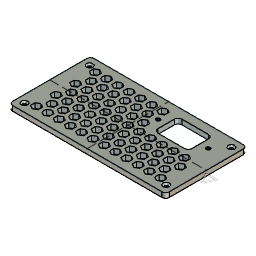
SFX+HDPLEX+Plate (Autodesk Fusion 360 design; units mm, degrees)
part number: 2025-09-21-12-47-08-713
Autodesk Fusion 360 part; units mm, degrees
sketch "Sketch1" plane through (0, 0, 0) normal (0, 0, 1) x (1, 0, 0)
  line L0 (59.5, 32.5) -> (-59.5, 32.5)
  line L1 (-62.5, 29.5) -> (-62.5, -29.5)
  line L2 (-59.5, -32.5) -> (59.5, -32.5)
  line L3 (62.5, -29.5) -> (62.5, 29.5)
  line L4 (62.5, 32.5) -> (-62.5, -32.5) construction
  line L5 (-62.5, 32.5) -> (62.5, -32.5) construction
  arc A0 (-59.5, 32.5) -> (-62.5, 29.5) centre (-59.5, 29.5) ccw
  arc A1 (62.5, 29.5) -> (59.5, 32.5) centre (59.5, 29.5) ccw
  arc A2 (-62.5, -29.5) -> (-59.5, -32.5) centre (-59.5, -29.5) ccw
  arc A3 (59.5, -32.5) -> (62.5, -29.5) centre (59.5, -29.5) ccw
  dimension "d1" = 125
  dimension "d2" = 65
  dimension "d3" = 3
  dimension "d4" = 3
  dimension "d5" = 3
  dimension "d6" = 3
  constraint horizontal L0
  constraint perpendicular L0 L1
  constraint parallel L0 L2
  constraint parallel L1 L3
  constraint coincident L4 origin
  constraint coincident L5 origin
  constraint coincident L5.start L1
  constraint coincident L5.start L0
  constraint tangent L1 A0
  constraint tangent L0 A0
  constraint coincident L4.start L0
  constraint coincident L4.start L3
  constraint tangent L0 A1
  constraint tangent L3 A1
  constraint coincident L4.end L1
  constraint coincident L4.end L2
  constraint tangent L1 A2
  constraint tangent L2 A2
  constraint coincident L5.end L2
  constraint coincident L5.end L3
  constraint tangent L2 A3
  constraint tangent L3 A3
  measures "d1" distance of L4.end L5.end
  measures "d2" distance of L5.start L4.end
  measures "d3" radius of A0
  measures "d4" radius of A1
  measures "d5" radius of A2
  measures "d6" radius of A3
extrude "Extrude1" add sketch "Sketch1" along normal blind 4
sketch "Sketch2" plane through (0, 0, 4) normal (0, 0, 1) x (-1, 0, 0)
  arc A0 (-59.5, 32.5) -> (-62.5, 29.5) centre (-59.5, 29.5) ccw
  line L0 (-62.5, 29.5) -> (-62.5, -29.5)
  arc A1 (-62.5, -29.5) -> (-59.5, -32.5) centre (-59.5, -29.5) ccw
  line L1 (-59.5, -32.5) -> (59.5, -32.5)
  arc A2 (59.5, -32.5) -> (62.5, -29.5) centre (59.5, -29.5) ccw
  line L2 (62.5, -29.5) -> (62.5, 29.5)
  arc A3 (62.5, 29.5) -> (59.5, 32.5) centre (59.5, 29.5) ccw
  line L3 (59.5, 32.5) -> (-59.5, 32.5)
  line L4 (0, 32.5) -> (0, -32.5) construction
  line L5 (62.5, 0) -> (-62.5, 0) construction
  constraint midpoint L3 L4.start
  constraint midpoint L1 L4.end
  constraint midpoint L2 L5.start
  constraint midpoint L0 L5.end
sketch "Sketch3" plane through (0, 0, 4) normal (0, 0, 1) x (1, 0, 0)
  line L0 (-62.5, 0) -> (62.5, 0)
  line L1 (0, -32.5) -> (0, 32.5)
  circle A0 centre (-56.5, -26) radius 1.75
  circle A1 centre (-56.5, 26) radius 1.75
  circle A2 centre (56.5, 26) radius 1.75
  circle A3 centre (56.5, -26) radius 1.75
  point P0 (-56.5, 26)
  point P1 (56.5, 26)
  point P2 (56.5, -26)
  point P3 (-56.5, -26)
  dimension "d10" = 56.5
  dimension "d11" = 26
  dimension "d12" = 56.5
  dimension "d13" = 26
  dimension "d14" = 56.5
  dimension "d15" = 26
  dimension "d17" = 26
  dimension "d18" = 56.5
  dimension "d19" = 3.5
  dimension "d20" = 3.5
  dimension "d21" = 3.5
  dimension "d22" = 3.5
  constraint coincident P3 A0.centre
  constraint coincident P0 A1.centre
  constraint coincident P1 A2.centre
  constraint coincident P2 A3.centre
  measures "d10" distance of P0 L1
  measures "d11" distance of P0 L0
  measures "d12" distance of L1 P1
  measures "d13" distance of L0 P1
  measures "d14" distance of L1 P2
  measures "d15" distance of L0 P2
  measures "d17" distance of L0 P3
  measures "d18" distance of L1 P3
  measures "d19" diameter of A0
  measures "d20" diameter of A1
  measures "d21" diameter of A2
  measures "d22" diameter of A3
hole "Hole1" at (-56.5, 26, 4) at (-56.5, -26, 4) at (56.5, 26, 4) at (56.5, -26, 4) direction (0, 0, -1) diameter 2.529 depth 4 tip angle 118 countersink diameter 5 countersink angle 90
thread "Thread1" "ISO Metric profile 3.0 M3x0.5 M3x0.5 6H" thread offset 0 thread depth 7.4
sketch "Sketch4" plane through (0, 0, 4) normal (0, 0, 1) x (-1, 0, 0)
  line L0 (-17.4, -25.6) -> (-38.6, -25.6)
  line L1 (-41.6, -22.6) -> (-41.6, -9.4)
  line L2 (-38.6, -6.4) -> (-17.4, -6.4)
  line L3 (-14.4, -9.4) -> (-14.4, -22.6)
  arc A0 (-17.4, -25.6) -> (-14.4, -22.6) centre (-17.4, -22.6) ccw
  arc A1 (-41.6, -22.6) -> (-38.6, -25.6) centre (-38.6, -22.6) ccw
  arc A2 (-14.4, -9.4) -> (-17.4, -6.4) centre (-17.4, -9.4) ccw
  arc A3 (-38.6, -6.4) -> (-41.6, -9.4) centre (-38.6, -9.4) ccw
  line L4 (0, 32.5) -> (0, -32.5)
  line L5 (62.5, 0) -> (-62.5, 0)
  circle A4 centre (-48, -16) radius 1
  circle A5 centre (-8, -16) radius 1
  point P0 (-14.4, -25.6)
  point P1 (-41.6, -25.6)
  point P2 (-14.4, -6.4)
  point P3 (-48, -16)
  point P4 (-8, -16)
  point P5 (-48, -16)
  dimension "d32" = 3
  dimension "d33" = 3
  dimension "d34" = 3
  dimension "d35" = 3
  dimension "d40" = 2
  dimension "d41" = 2
  constraint coincident P0 L3
  constraint coincident P0 L0
  constraint tangent L3 A0
  constraint tangent L0 A0
  constraint coincident P1 L0
  constraint coincident P1 L1
  constraint tangent L0 A1
  constraint tangent L1 A1
  constraint coincident P2 L2
  constraint coincident P2 L3
  constraint tangent L2 A2
  constraint tangent L3 A2
  constraint tangent L2 A3
  constraint tangent L1 A3
  constraint coincident P5 P3
  constraint coincident P4 A5.centre
  measures "d32" radius of A0
  measures "d33" radius of A1
  measures "d34" radius of A2
  measures "d35" radius of A3
  measures "d40" diameter of A4
  measures "d41" diameter of A5
extrude "Extrude2" cut sketch "Sketch4" against normal blind 4
sketch "Sketch5" plane through (0, 0, 4) normal (0, 0, 1) x (-1, 0, 0)
  point P0 (-48, -16)
  point P1 (-8, -16)
hole "Hole2" at (48, 16, 4) at (8, 16, 4) direction (0, 0, -1) diameter 2.529 depth 4 tip angle 118
thread "Thread2" "ISO Metric profile 3.0 M3x0.5 M3x0.5 6H" thread offset 0 thread depth 7.4
sketch "Sketch6" plane through (0, 0, 4) normal (0, 0, 1) x (-1, 0, 0)
  line L0 (-3, -1.7321) -> (0, -3.4641)
  line L1 (0, -3.4641) -> (3, -1.7321)
  line L2 (3, -1.7321) -> (3, 1.7321)
  line L3 (3, 1.7321) -> (0, 3.4641)
  line L4 (0, 3.4641) -> (-3, 1.7321)
  line L5 (-3, 1.7321) -> (-3, -1.7321)
  line L6 (-48, -1.7321) -> (-45, -3.4641)
  line L7 (-45, -3.4641) -> (-42, -1.7321)
  line L8 (-42, -1.7321) -> (-42, 1.7321)
  line L9 (-42, 1.7321) -> (-45, 3.4641)
  line L10 (-48, 1.7321) -> (-48, -1.7321)
  line L11 (-45, 3.4641) -> (-48, 1.7321)
  line L12 (-39, -1.7321) -> (-36, -3.4641)
  line L13 (-36, -3.4641) -> (-33, -1.7321)
  line L14 (-33, -1.7321) -> (-33, 1.7321)
  line L15 (-33, 1.7321) -> (-36, 3.4641)
  line L16 (-39, 1.7321) -> (-39, -1.7321)
  line L17 (-36, 3.4641) -> (-39, 1.7321)
  line L18 (-30, -1.7321) -> (-27, -3.4641)
  line L19 (-27, -3.4641) -> (-24, -1.7321)
  line L20 (-24, -1.7321) -> (-24, 1.7321)
  line L21 (-24, 1.7321) -> (-27, 3.4641)
  line L22 (-30, 1.7321) -> (-30, -1.7321)
  line L23 (-27, 3.4641) -> (-30, 1.7321)
  line L24 (-21, -1.7321) -> (-18, -3.4641)
  line L25 (-18, -3.4641) -> (-15, -1.7321)
  line L26 (-15, -1.7321) -> (-15, 1.7321)
  line L27 (-15, 1.7321) -> (-18, 3.4641)
  line L28 (-21, 1.7321) -> (-21, -1.7321)
  line L29 (-18, 3.4641) -> (-21, 1.7321)
  line L30 (-12, -1.7321) -> (-9, -3.4641)
  line L31 (-9, -3.4641) -> (-6, -1.7321)
  line L32 (-6, -1.7321) -> (-6, 1.7321)
  line L33 (-6, 1.7321) -> (-9, 3.4641)
  line L34 (-12, 1.7321) -> (-12, -1.7321)
  line L35 (-9, 3.4641) -> (-12, 1.7321)
  line L36 (6, -1.7321) -> (9, -3.4641)
  line L37 (9, -3.4641) -> (12, -1.7321)
  line L38 (12, -1.7321) -> (12, 1.7321)
  line L39 (12, 1.7321) -> (9, 3.4641)
  line L40 (6, 1.7321) -> (6, -1.7321)
  line L41 (9, 3.4641) -> (6, 1.7321)
  line L42 (15, -1.7321) -> (18, -3.4641)
  line L43 (18, -3.4641) -> (21, -1.7321)
  line L44 (21, -1.7321) -> (21, 1.7321)
  line L45 (21, 1.7321) -> (18, 3.4641)
  line L46 (15, 1.7321) -> (15, -1.7321)
  line L47 (18, 3.4641) -> (15, 1.7321)
  line L48 (24, -1.7321) -> (27, -3.4641)
  line L49 (27, -3.4641) -> (30, -1.7321)
  line L50 (30, -1.7321) -> (30, 1.7321)
  line L51 (30, 1.7321) -> (27, 3.4641)
  line L52 (24, 1.7321) -> (24, -1.7321)
  line L53 (27, 3.4641) -> (24, 1.7321)
  line L54 (33, -1.7321) -> (36, -3.4641)
  line L55 (36, -3.4641) -> (39, -1.7321)
  line L56 (39, -1.7321) -> (39, 1.7321)
  line L57 (39, 1.7321) -> (36, 3.4641)
  line L58 (33, 1.7321) -> (33, -1.7321)
  line L59 (36, 3.4641) -> (33, 1.7321)
  line L60 (42, -1.7321) -> (45, -3.4641)
  line L61 (45, -3.4641) -> (48, -1.7321)
  line L62 (48, -1.7321) -> (48, 1.7321)
  line L63 (48, 1.7321) -> (45, 3.4641)
  line L64 (42, 1.7321) -> (42, -1.7321)
  line L65 (45, 3.4641) -> (42, 1.7321)
  line L66 (48, -1.7321) -> (48, 1.7321)
  line L67 (48, 1.7321) -> (45, 3.4641)
  line L68 (45, 3.4641) -> (42, 1.7321)
  line L69 (42, 1.7321) -> (42, -1.7321)
  line L70 (42, -1.7321) -> (45, -3.4641)
  line L71 (45, -3.4641) -> (48, -1.7321)
  line L72 (39, -1.7321) -> (39, 1.7321)
  line L73 (39, 1.7321) -> (36, 3.4641)
  line L74 (36, 3.4641) -> (33, 1.7321)
  line L75 (33, 1.7321) -> (33, -1.7321)
  line L76 (36, -3.4641) -> (39, -1.7321)
  line L77 (33, -1.7321) -> (36, -3.4641)
  line L78 (30, -1.7321) -> (30, 1.7321)
  line L79 (30, 1.7321) -> (27, 3.4641)
  line L80 (27, 3.4641) -> (24, 1.7321)
  line L81 (24, 1.7321) -> (24, -1.7321)
  line L82 (27, -3.4641) -> (30, -1.7321)
  line L83 (24, -1.7321) -> (27, -3.4641)
  line L84 (21, -1.7321) -> (21, 1.7321)
  line L85 (21, 1.7321) -> (18, 3.4641)
  line L86 (18, 3.4641) -> (15, 1.7321)
  line L87 (15, 1.7321) -> (15, -1.7321)
  line L88 (18, -3.4641) -> (21, -1.7321)
  line L89 (15, -1.7321) -> (18, -3.4641)
  line L90 (12, -1.7321) -> (12, 1.7321)
  line L91 (12, 1.7321) -> (9, 3.4641)
  line L92 (9, 3.4641) -> (6, 1.7321)
  line L93 (6, 1.7321) -> (6, -1.7321)
  line L94 (9, -3.4641) -> (12, -1.7321)
  line L95 (6, -1.7321) -> (9, -3.4641)
  line L96 (3, -1.7321) -> (3, 1.7321)
  line L97 (3, 1.7321) -> (0, 3.4641)
  line L98 (0, 3.4641) -> (-3, 1.7321)
  line L99 (-3, 1.7321) -> (-3, -1.7321)
  line L100 (0, -3.4641) -> (3, -1.7321)
  line L101 (-3, -1.7321) -> (0, -3.4641)
  line L102 (-6, -1.7321) -> (-6, 1.7321)
  line L103 (-6, 1.7321) -> (-9, 3.4641)
  line L104 (-9, 3.4641) -> (-12, 1.7321)
  line L105 (-12, 1.7321) -> (-12, -1.7321)
  line L106 (-9, -3.4641) -> (-6, -1.7321)
  line L107 (-12, -1.7321) -> (-9, -3.4641)
  line L108 (-15, -1.7321) -> (-15, 1.7321)
  line L109 (-15, 1.7321) -> (-18, 3.4641)
  line L110 (-18, 3.4641) -> (-21, 1.7321)
  line L111 (-21, 1.7321) -> (-21, -1.7321)
  line L112 (-18, -3.4641) -> (-15, -1.7321)
  line L113 (-21, -1.7321) -> (-18, -3.4641)
  line L114 (-24, -1.7321) -> (-24, 1.7321)
  line L115 (-24, 1.7321) -> (-27, 3.4641)
  line L116 (-27, 3.4641) -> (-30, 1.7321)
  line L117 (-30, 1.7321) -> (-30, -1.7321)
  line L118 (-27, -3.4641) -> (-24, -1.7321)
  line L119 (-30, -1.7321) -> (-27, -3.4641)
  line L120 (-33, -1.7321) -> (-33, 1.7321)
  line L121 (-33, 1.7321) -> (-36, 3.4641)
  line L122 (-36, 3.4641) -> (-39, 1.7321)
  line L123 (-39, 1.7321) -> (-39, -1.7321)
  line L124 (-36, -3.4641) -> (-33, -1.7321)
  line L125 (-39, -1.7321) -> (-36, -3.4641)
  line L126 (-42, -1.7321) -> (-42, 1.7321)
  line L127 (-42, 1.7321) -> (-45, 3.4641)
  line L128 (-45, 3.4641) -> (-48, 1.7321)
  line L129 (-48, 1.7321) -> (-48, -1.7321)
  line L130 (-45, -3.4641) -> (-42, -1.7321)
  line L131 (-48, -1.7321) -> (-45, -3.4641)
  line L132 (48, -1.7321) -> (48, 1.7321)
  line L133 (48, 1.7321) -> (45, 3.4641)
  line L134 (45, 3.4641) -> (42, 1.7321)
  line L135 (42, 1.7321) -> (42, -1.7321)
  line L136 (42, -1.7321) -> (45, -3.4641)
  line L137 (45, -3.4641) -> (48, -1.7321)
  line L138 (39, -1.7321) -> (39, 1.7321)
  line L139 (39, 1.7321) -> (36, 3.4641)
  line L140 (36, 3.4641) -> (33, 1.7321)
  line L141 (33, 1.7321) -> (33, -1.7321)
  line L142 (36, -3.4641) -> (39, -1.7321)
  line L143 (33, -1.7321) -> (36, -3.4641)
  line L144 (30, -1.7321) -> (30, 1.7321)
  line L145 (30, 1.7321) -> (27, 3.4641)
  line L146 (27, 3.4641) -> (24, 1.7321)
  line L147 (24, 1.7321) -> (24, -1.7321)
  line L148 (27, -3.4641) -> (30, -1.7321)
  line L149 (24, -1.7321) -> (27, -3.4641)
  line L150 (21, -1.7321) -> (21, 1.7321)
  line L151 (21, 1.7321) -> (18, 3.4641)
  line L152 (18, 3.4641) -> (15, 1.7321)
  line L153 (15, 1.7321) -> (15, -1.7321)
  line L154 (18, -3.4641) -> (21, -1.7321)
  line L155 (15, -1.7321) -> (18, -3.4641)
  line L156 (12, -1.7321) -> (12, 1.7321)
  line L157 (12, 1.7321) -> (9, 3.4641)
  line L158 (9, 3.4641) -> (6, 1.7321)
  line L159 (6, 1.7321) -> (6, -1.7321)
  line L160 (9, -3.4641) -> (12, -1.7321)
  line L161 (6, -1.7321) -> (9, -3.4641)
  line L162 (3, -1.7321) -> (3, 1.7321)
  line L163 (3, 1.7321) -> (0, 3.4641)
  line L164 (0, 3.4641) -> (-3, 1.7321)
  line L165 (-3, 1.7321) -> (-3, -1.7321)
  line L166 (0, -3.4641) -> (3, -1.7321)
  line L167 (-3, -1.7321) -> (0, -3.4641)
  line L168 (-6, -1.7321) -> (-6, 1.7321)
  line L169 (-6, 1.7321) -> (-9, 3.4641)
  line L170 (-9, 3.4641) -> (-12, 1.7321)
  line L171 (-12, 1.7321) -> (-12, -1.7321)
  line L172 (-9, -3.4641) -> (-6, -1.7321)
  line L173 (-12, -1.7321) -> (-9, -3.4641)
  line L174 (-15, -1.7321) -> (-15, 1.7321)
  line L175 (-15, 1.7321) -> (-18, 3.4641)
  line L176 (-18, 3.4641) -> (-21, 1.7321)
  line L177 (-21, 1.7321) -> (-21, -1.7321)
  line L178 (-18, -3.4641) -> (-15, -1.7321)
  line L179 (-21, -1.7321) -> (-18, -3.4641)
  line L180 (-24, -1.7321) -> (-24, 1.7321)
  line L181 (-24, 1.7321) -> (-27, 3.4641)
  line L182 (-27, 3.4641) -> (-30, 1.7321)
  line L183 (-30, 1.7321) -> (-30, -1.7321)
  line L184 (-27, -3.4641) -> (-24, -1.7321)
  line L185 (-30, -1.7321) -> (-27, -3.4641)
  line L186 (-33, -1.7321) -> (-33, 1.7321)
  line L187 (-33, 1.7321) -> (-36, 3.4641)
  line L188 (-36, 3.4641) -> (-39, 1.7321)
  line L189 (-39, 1.7321) -> (-39, -1.7321)
  line L190 (-36, -3.4641) -> (-33, -1.7321)
  line L191 (-39, -1.7321) -> (-36, -3.4641)
  line L192 (-42, -1.7321) -> (-42, 1.7321)
  line L193 (-42, 1.7321) -> (-45, 3.4641)
  line L194 (-45, 3.4641) -> (-48, 1.7321)
  line L195 (-48, 1.7321) -> (-48, -1.7321)
  line L196 (-45, -3.4641) -> (-42, -1.7321)
  line L197 (-48, -1.7321) -> (-45, -3.4641)
  line L198 (48, -1.7321) -> (48, 1.7321)
  line L199 (48, 1.7321) -> (45, 3.4641)
  line L200 (45, 3.4641) -> (42, 1.7321)
  line L201 (42, 1.7321) -> (42, -1.7321)
  line L202 (42, -1.7321) -> (45, -3.4641)
  line L203 (45, -3.4641) -> (48, -1.7321)
  line L204 (39, -1.7321) -> (39, 1.7321)
  line L205 (39, 1.7321) -> (36, 3.4641)
  line L206 (36, 3.4641) -> (33, 1.7321)
  line L207 (33, 1.7321) -> (33, -1.7321)
  line L208 (36, -3.4641) -> (39, -1.7321)
  line L209 (33, -1.7321) -> (36, -3.4641)
  line L210 (30, -1.7321) -> (30, 1.7321)
  line L211 (30, 1.7321) -> (27, 3.4641)
  line L212 (27, 3.4641) -> (24, 1.7321)
  line L213 (24, 1.7321) -> (24, -1.7321)
  line L214 (27, -3.4641) -> (30, -1.7321)
  line L215 (24, -1.7321) -> (27, -3.4641)
  line L216 (21, -1.7321) -> (21, 1.7321)
  line L217 (21, 1.7321) -> (18, 3.4641)
  line L218 (18, 3.4641) -> (15, 1.7321)
  line L219 (15, 1.7321) -> (15, -1.7321)
  line L220 (18, -3.4641) -> (21, -1.7321)
  line L221 (15, -1.7321) -> (18, -3.4641)
  line L222 (12, -1.7321) -> (12, 1.7321)
  line L223 (12, 1.7321) -> (9, 3.4641)
  line L224 (9, 3.4641) -> (6, 1.7321)
  line L225 (6, 1.7321) -> (6, -1.7321)
  line L226 (9, -3.4641) -> (12, -1.7321)
  line L227 (6, -1.7321) -> (9, -3.4641)
  line L228 (3, -1.7321) -> (3, 1.7321)
  line L229 (3, 1.7321) -> (0, 3.4641)
  line L230 (0, 3.4641) -> (-3, 1.7321)
  line L231 (-3, 1.7321) -> (-3, -1.7321)
  line L232 (0, -3.4641) -> (3, -1.7321)
  line L233 (-3, -1.7321) -> (0, -3.4641)
  line L234 (-6, -1.7321) -> (-6, 1.7321)
  line L235 (-6, 1.7321) -> (-9, 3.4641)
  line L236 (-9, 3.4641) -> (-12, 1.7321)
  line L237 (-12, 1.7321) -> (-12, -1.7321)
  line L238 (-9, -3.4641) -> (-6, -1.7321)
  line L239 (-12, -1.7321) -> (-9, -3.4641)
  line L240 (-15, -1.7321) -> (-15, 1.7321)
  line L241 (-15, 1.7321) -> (-18, 3.4641)
  line L242 (-18, 3.4641) -> (-21, 1.7321)
  line L243 (-21, 1.7321) -> (-21, -1.7321)
  line L244 (-18, -3.4641) -> (-15, -1.7321)
  line L245 (-21, -1.7321) -> (-18, -3.4641)
  line L246 (-24, -1.7321) -> (-24, 1.7321)
  line L247 (-24, 1.7321) -> (-27, 3.4641)
  line L248 (-27, 3.4641) -> (-30, 1.7321)
  line L249 (-30, 1.7321) -> (-30, -1.7321)
  line L250 (-27, -3.4641) -> (-24, -1.7321)
  line L251 (-30, -1.7321) -> (-27, -3.4641)
  line L252 (-33, -1.7321) -> (-33, 1.7321)
  line L253 (-33, 1.7321) -> (-36, 3.4641)
  line L254 (-36, 3.4641) -> (-39, 1.7321)
  line L255 (-39, 1.7321) -> (-39, -1.7321)
  line L256 (-36, -3.4641) -> (-33, -1.7321)
  line L257 (-39, -1.7321) -> (-36, -3.4641)
  line L258 (-42, -1.7321) -> (-42, 1.7321)
  line L259 (-42, 1.7321) -> (-45, 3.4641)
  line L260 (-45, 3.4641) -> (-48, 1.7321)
  line L261 (-48, 1.7321) -> (-48, -1.7321)
  line L262 (-45, -3.4641) -> (-42, -1.7321)
  line L263 (-48, -1.7321) -> (-45, -3.4641)
  line L264 (-30, 1.7321) -> (-30, -1.7321)
  line L265 (-30, -1.7321) -> (-27, -3.4641)
  line L266 (-27, -3.4641) -> (-24, -1.7321)
  line L267 (-24, -1.7321) -> (-24, 1.7321)
  line L268 (-27, 3.4641) -> (-30, 1.7321)
  line L269 (-24, 1.7321) -> (-27, 3.4641)
  line L270 (-39, 1.7321) -> (-39, -1.7321)
  line L271 (-39, -1.7321) -> (-36, -3.4641)
  line L272 (-36, -3.4641) -> (-33, -1.7321)
  line L273 (-33, -1.7321) -> (-33, 1.7321)
  line L274 (-36, 3.4641) -> (-39, 1.7321)
  line L275 (-33, 1.7321) -> (-36, 3.4641)
  line L276 (-48, 1.7321) -> (-48, -1.7321)
  line L277 (-48, -1.7321) -> (-45, -3.4641)
  line L278 (-45, -3.4641) -> (-42, -1.7321)
  line L279 (-42, -1.7321) -> (-42, 1.7321)
  line L280 (-45, 3.4641) -> (-48, 1.7321)
  line L281 (-42, 1.7321) -> (-45, 3.4641)
  line L282 (-21, 1.7321) -> (-21, -1.7321)
  line L283 (-21, -1.7321) -> (-18, -3.4641)
  line L284 (-18, -3.4641) -> (-15, -1.7321)
  line L285 (-15, -1.7321) -> (-15, 1.7321)
  line L286 (-18, 3.4641) -> (-21, 1.7321)
  line L287 (-15, 1.7321) -> (-18, 3.4641)
  line L288 (-12, 1.7321) -> (-12, -1.7321)
  line L289 (-12, -1.7321) -> (-9, -3.4641)
  line L290 (-9, -3.4641) -> (-6, -1.7321)
  line L291 (-6, -1.7321) -> (-6, 1.7321)
  line L292 (-9, 3.4641) -> (-12, 1.7321)
  line L293 (-6, 1.7321) -> (-9, 3.4641)
  line L294 (-3, 1.7321) -> (-3, -1.7321)
  line L295 (-3, -1.7321) -> (0, -3.4641)
  line L296 (0, -3.4641) -> (3, -1.7321)
  line L297 (3, -1.7321) -> (3, 1.7321)
  line L298 (0, 3.4641) -> (-3, 1.7321)
  line L299 (3, 1.7321) -> (0, 3.4641)
  line L300 (6, 1.7321) -> (6, -1.7321)
  line L301 (6, -1.7321) -> (9, -3.4641)
  line L302 (9, -3.4641) -> (12, -1.7321)
  line L303 (12, -1.7321) -> (12, 1.7321)
  line L304 (9, 3.4641) -> (6, 1.7321)
  line L305 (12, 1.7321) -> (9, 3.4641)
  line L306 (15, 1.7321) -> (15, -1.7321)
  line L307 (15, -1.7321) -> (18, -3.4641)
  line L308 (18, -3.4641) -> (21, -1.7321)
  line L309 (21, -1.7321) -> (21, 1.7321)
  line L310 (18, 3.4641) -> (15, 1.7321)
  line L311 (21, 1.7321) -> (18, 3.4641)
  line L312 (24, 1.7321) -> (24, -1.7321)
  line L313 (24, -1.7321) -> (27, -3.4641)
  line L314 (27, -3.4641) -> (30, -1.7321)
  line L315 (30, -1.7321) -> (30, 1.7321)
  line L316 (27, 3.4641) -> (24, 1.7321)
  line L317 (30, 1.7321) -> (27, 3.4641)
  line L318 (33, 1.7321) -> (33, -1.7321)
  line L319 (33, -1.7321) -> (36, -3.4641)
  line L320 (36, -3.4641) -> (39, -1.7321)
  line L321 (39, -1.7321) -> (39, 1.7321)
  line L322 (36, 3.4641) -> (33, 1.7321)
  line L323 (39, 1.7321) -> (36, 3.4641)
  line L324 (42, 1.7321) -> (42, -1.7321)
  line L325 (42, -1.7321) -> (45, -3.4641)
  line L326 (45, -3.4641) -> (48, -1.7321)
  line L327 (48, -1.7321) -> (48, 1.7321)
  line L328 (45, 3.4641) -> (42, 1.7321)
  line L329 (48, 1.7321) -> (45, 3.4641)
  line L330 (-30, 1.7321) -> (-30, -1.7321)
  line L331 (-30, -1.7321) -> (-27, -3.4641)
  line L332 (-27, -3.4641) -> (-24, -1.7321)
  line L333 (-24, -1.7321) -> (-24, 1.7321)
  line L334 (-27, 3.4641) -> (-30, 1.7321)
  line L335 (-24, 1.7321) -> (-27, 3.4641)
  line L336 (-39, 1.7321) -> (-39, -1.7321)
  line L337 (-39, -1.7321) -> (-36, -3.4641)
  line L338 (-36, -3.4641) -> (-33, -1.7321)
  line L339 (-33, -1.7321) -> (-33, 1.7321)
  line L340 (-36, 3.4641) -> (-39, 1.7321)
  line L341 (-33, 1.7321) -> (-36, 3.4641)
  line L342 (-48, 1.7321) -> (-48, -1.7321)
  line L343 (-48, -1.7321) -> (-45, -3.4641)
  line L344 (-45, -3.4641) -> (-42, -1.7321)
  line L345 (-42, -1.7321) -> (-42, 1.7321)
  line L346 (-45, 3.4641) -> (-48, 1.7321)
  line L347 (-42, 1.7321) -> (-45, 3.4641)
  line L348 (-21, 1.7321) -> (-21, -1.7321)
  line L349 (-21, -1.7321) -> (-18, -3.4641)
  line L350 (-18, -3.4641) -> (-15, -1.7321)
  line L351 (-15, -1.7321) -> (-15, 1.7321)
  line L352 (-18, 3.4641) -> (-21, 1.7321)
  line L353 (-15, 1.7321) -> (-18, 3.4641)
  line L354 (-12, 1.7321) -> (-12, -1.7321)
  line L355 (-12, -1.7321) -> (-9, -3.4641)
  line L356 (-9, -3.4641) -> (-6, -1.7321)
  line L357 (-6, -1.7321) -> (-6, 1.7321)
  line L358 (-9, 3.4641) -> (-12, 1.7321)
  line L359 (-6, 1.7321) -> (-9, 3.4641)
  line L360 (-3, 1.7321) -> (-3, -1.7321)
  line L361 (-3, -1.7321) -> (0, -3.4641)
  line L362 (0, -3.4641) -> (3, -1.7321)
  line L363 (3, -1.7321) -> (3, 1.7321)
  line L364 (0, 3.4641) -> (-3, 1.7321)
  line L365 (3, 1.7321) -> (0, 3.4641)
  line L366 (6, 1.7321) -> (6, -1.7321)
  line L367 (6, -1.7321) -> (9, -3.4641)
  line L368 (9, -3.4641) -> (12, -1.7321)
  line L369 (12, -1.7321) -> (12, 1.7321)
  line L370 (9, 3.4641) -> (6, 1.7321)
  line L371 (12, 1.7321) -> (9, 3.4641)
  line L372 (15, 1.7321) -> (15, -1.7321)
  line L373 (15, -1.7321) -> (18, -3.4641)
  line L374 (18, -3.4641) -> (21, -1.7321)
  line L375 (21, -1.7321) -> (21, 1.7321)
  line L376 (18, 3.4641) -> (15, 1.7321)
  line L377 (21, 1.7321) -> (18, 3.4641)
  line L378 (24, 1.7321) -> (24, -1.7321)
  line L379 (24, -1.7321) -> (27, -3.4641)
  line L380 (27, -3.4641) -> (30, -1.7321)
  line L381 (30, -1.7321) -> (30, 1.7321)
  line L382 (27, 3.4641) -> (24, 1.7321)
  line L383 (30, 1.7321) -> (27, 3.4641)
  line L384 (33, 1.7321) -> (33, -1.7321)
  line L385 (33, -1.7321) -> (36, -3.4641)
  line L386 (36, -3.4641) -> (39, -1.7321)
  line L387 (39, -1.7321) -> (39, 1.7321)
  line L388 (36, 3.4641) -> (33, 1.7321)
  line L389 (39, 1.7321) -> (36, 3.4641)
  line L390 (42, 1.7321) -> (42, -1.7321)
  line L391 (42, -1.7321) -> (45, -3.4641)
  line L392 (45, -3.4641) -> (48, -1.7321)
  line L393 (48, -1.7321) -> (48, 1.7321)
  line L394 (45, 3.4641) -> (42, 1.7321)
  line L395 (48, 1.7321) -> (45, 3.4641)
  line L396 (-25.5, 9.5321) -> (-25.5, 6.0679)
  line L397 (-25.5, 6.0679) -> (-22.5, 4.3359)
  line L398 (-22.5, 4.3359) -> (-19.5, 6.0679)
  line L399 (-19.5, 6.0679) -> (-19.5, 9.5321)
  line L400 (-22.5, 11.2641) -> (-25.5, 9.5321)
  line L401 (-19.5, 9.5321) -> (-22.5, 11.2641)
  line L402 (-34.5, 9.5321) -> (-34.5, 6.0679)
  line L403 (-34.5, 6.0679) -> (-31.5, 4.3359)
  line L404 (-31.5, 4.3359) -> (-28.5, 6.0679)
  line L405 (-28.5, 6.0679) -> (-28.5, 9.5321)
  line L406 (-31.5, 11.2641) -> (-34.5, 9.5321)
  line L407 (-28.5, 9.5321) -> (-31.5, 11.2641)
  line L408 (-43.5, 9.5321) -> (-43.5, 6.0679)
  line L409 (-43.5, 6.0679) -> (-40.5, 4.3359)
  line L410 (-40.5, 4.3359) -> (-37.5, 6.0679)
  line L411 (-37.5, 6.0679) -> (-37.5, 9.5321)
  line L412 (-40.5, 11.2641) -> (-43.5, 9.5321)
  line L413 (-37.5, 9.5321) -> (-40.5, 11.2641)
  line L414 (-16.5, 9.5321) -> (-16.5, 6.0679)
  line L415 (-16.5, 6.0679) -> (-13.5, 4.3359)
  line L416 (-13.5, 4.3359) -> (-10.5, 6.0679)
  line L417 (-10.5, 6.0679) -> (-10.5, 9.5321)
  line L418 (-13.5, 11.2641) -> (-16.5, 9.5321)
  line L419 (-10.5, 9.5321) -> (-13.5, 11.2641)
  line L420 (-7.5, 9.5321) -> (-7.5, 6.0679)
  line L421 (-7.5, 6.0679) -> (-4.5, 4.3359)
  line L422 (-4.5, 4.3359) -> (-1.5, 6.0679)
  line L423 (-1.5, 6.0679) -> (-1.5, 9.5321)
  line L424 (-4.5, 11.2641) -> (-7.5, 9.5321)
  line L425 (-1.5, 9.5321) -> (-4.5, 11.2641)
  line L426 (1.5, 9.5321) -> (1.5, 6.0679)
  line L427 (1.5, 6.0679) -> (4.5, 4.3359)
  line L428 (4.5, 4.3359) -> (7.5, 6.0679)
  line L429 (7.5, 6.0679) -> (7.5, 9.5321)
  line L430 (4.5, 11.2641) -> (1.5, 9.5321)
  line L431 (7.5, 9.5321) -> (4.5, 11.2641)
  line L432 (10.5, 9.5321) -> (10.5, 6.0679)
  line L433 (10.5, 6.0679) -> (13.5, 4.3359)
  line L434 (13.5, 4.3359) -> (16.5, 6.0679)
  line L435 (16.5, 6.0679) -> (16.5, 9.5321)
  line L436 (13.5, 11.2641) -> (10.5, 9.5321)
  line L437 (16.5, 9.5321) -> (13.5, 11.2641)
  line L438 (19.5, 9.5321) -> (19.5, 6.0679)
  line L439 (19.5, 6.0679) -> (22.5, 4.3359)
  line L440 (22.5, 4.3359) -> (25.5, 6.0679)
  line L441 (25.5, 6.0679) -> (25.5, 9.5321)
  line L442 (22.5, 11.2641) -> (19.5, 9.5321)
  line L443 (25.5, 9.5321) -> (22.5, 11.2641)
  line L444 (28.5, 9.5321) -> (28.5, 6.0679)
  line L445 (28.5, 6.0679) -> (31.5, 4.3359)
  line L446 (31.5, 4.3359) -> (34.5, 6.0679)
  line L447 (34.5, 6.0679) -> (34.5, 9.5321)
  line L448 (31.5, 11.2641) -> (28.5, 9.5321)
  line L449 (34.5, 9.5321) -> (31.5, 11.2641)
  line L450 (37.5, 9.5321) -> (37.5, 6.0679)
  line L451 (37.5, 6.0679) -> (40.5, 4.3359)
  line L452 (40.5, 4.3359) -> (43.5, 6.0679)
  line L453 (43.5, 6.0679) -> (43.5, 9.5321)
  line L454 (40.5, 11.2641) -> (37.5, 9.5321)
  line L455 (43.5, 9.5321) -> (40.5, 11.2641)
  line L456 (46.5, 9.5321) -> (46.5, 6.0679)
  line L457 (46.5, 6.0679) -> (49.5, 4.3359)
  line L458 (49.5, 4.3359) -> (52.5, 6.0679)
  line L459 (52.5, 6.0679) -> (52.5, 9.5321)
  line L460 (49.5, 11.2641) -> (46.5, 9.5321)
  line L461 (52.5, 9.5321) -> (49.5, 11.2641)
  line L462 (-52.5, 6.0679) -> (-49.5, 4.3359)
  line L463 (-49.5, 4.3359) -> (-46.5, 6.0679)
  line L464 (-46.5, 6.0679) -> (-46.5, 9.5321)
  line L465 (-46.5, 9.5321) -> (-49.5, 11.2641)
  line L466 (-49.5, 11.2641) -> (-52.5, 9.5321)
  line L467 (-52.5, 9.5321) -> (-52.5, 6.0679)
  line L468 (-7.5, -6.0679) -> (-7.5, -9.5321)
  line L469 (-7.5, -9.5321) -> (-4.5, -11.2641)
  line L470 (-4.5, -11.2641) -> (-1.5, -9.5321)
  line L471 (-1.5, -9.5321) -> (-1.5, -6.0679)
  line L472 (-4.5, -4.3359) -> (-7.5, -6.0679)
  line L473 (-1.5, -6.0679) -> (-4.5, -4.3359)
  line L474 (1.5, -6.0679) -> (1.5, -9.5321)
  line L475 (1.5, -9.5321) -> (4.5, -11.2641)
  line L476 (4.5, -11.2641) -> (7.5, -9.5321)
  line L477 (7.5, -9.5321) -> (7.5, -6.0679)
  line L478 (4.5, -4.3359) -> (1.5, -6.0679)
  line L479 (7.5, -6.0679) -> (4.5, -4.3359)
  line L480 (10.5, -6.0679) -> (10.5, -9.5321)
  line L481 (10.5, -9.5321) -> (13.5, -11.2641)
  line L482 (13.5, -11.2641) -> (16.5, -9.5321)
  line L483 (16.5, -9.5321) -> (16.5, -6.0679)
  line L484 (13.5, -4.3359) -> (10.5, -6.0679)
  line L485 (16.5, -6.0679) -> (13.5, -4.3359)
  line L486 (19.5, -6.0679) -> (19.5, -9.5321)
  line L487 (19.5, -9.5321) -> (22.5, -11.2641)
  line L488 (22.5, -11.2641) -> (25.5, -9.5321)
  line L489 (25.5, -9.5321) -> (25.5, -6.0679)
  line L490 (22.5, -4.3359) -> (19.5, -6.0679)
  line L491 (25.5, -6.0679) -> (22.5, -4.3359)
  line L492 (28.5, -6.0679) -> (28.5, -9.5321)
  line L493 (28.5, -9.5321) -> (31.5, -11.2641)
  line L494 (31.5, -11.2641) -> (34.5, -9.5321)
  line L495 (34.5, -9.5321) -> (34.5, -6.0679)
  line L496 (31.5, -4.3359) -> (28.5, -6.0679)
  line L497 (34.5, -6.0679) -> (31.5, -4.3359)
  line L498 (37.5, -6.0679) -> (37.5, -9.5321)
  line L499 (37.5, -9.5321) -> (40.5, -11.2641)
  line L500 (40.5, -11.2641) -> (43.5, -9.5321)
  line L501 (43.5, -9.5321) -> (43.5, -6.0679)
  line L502 (40.5, -4.3359) -> (37.5, -6.0679)
  line L503 (43.5, -6.0679) -> (40.5, -4.3359)
  line L504 (46.5, -6.0679) -> (46.5, -9.5321)
  line L505 (46.5, -9.5321) -> (49.5, -11.2641)
  line L506 (49.5, -11.2641) -> (52.5, -9.5321)
  line L507 (52.5, -9.5321) -> (52.5, -6.0679)
  line L508 (49.5, -4.3359) -> (46.5, -6.0679)
  line L509 (52.5, -6.0679) -> (49.5, -4.3359)
  line L510 (-30, 17.3321) -> (-30, 13.8679)
  line L511 (-30, 13.8679) -> (-27, 12.1359)
  line L512 (-27, 12.1359) -> (-24, 13.8679)
  line L513 (-24, 13.8679) -> (-24, 17.3321)
  line L514 (-27, 19.0641) -> (-30, 17.3321)
  line L515 (-24, 17.3321) -> (-27, 19.0641)
  line L516 (-39, 17.3321) -> (-39, 13.8679)
  line L517 (-39, 13.8679) -> (-36, 12.1359)
  line L518 (-36, 12.1359) -> (-33, 13.8679)
  line L519 (-33, 13.8679) -> (-33, 17.3321)
  line L520 (-36, 19.0641) -> (-39, 17.3321)
  line L521 (-33, 17.3321) -> (-36, 19.0641)
  line L522 (-48, 17.3321) -> (-48, 13.8679)
  line L523 (-48, 13.8679) -> (-45, 12.1359)
  line L524 (-45, 12.1359) -> (-42, 13.8679)
  line L525 (-42, 13.8679) -> (-42, 17.3321)
  line L526 (-45, 19.0641) -> (-48, 17.3321)
  line L527 (-42, 17.3321) -> (-45, 19.0641)
  line L528 (-21, 17.3321) -> (-21, 13.8679)
  line L529 (-21, 13.8679) -> (-18, 12.1359)
  line L530 (-18, 12.1359) -> (-15, 13.8679)
  line L531 (-15, 13.8679) -> (-15, 17.3321)
  line L532 (-18, 19.0641) -> (-21, 17.3321)
  line L533 (-15, 17.3321) -> (-18, 19.0641)
  line L534 (-12, 17.3321) -> (-12, 13.8679)
  line L535 (-12, 13.8679) -> (-9, 12.1359)
  line L536 (-9, 12.1359) -> (-6, 13.8679)
  line L537 (-6, 13.8679) -> (-6, 17.3321)
  line L538 (-9, 19.0641) -> (-12, 17.3321)
  line L539 (-6, 17.3321) -> (-9, 19.0641)
  line L540 (-3, 17.3321) -> (-3, 13.8679)
  line L541 (-3, 13.8679) -> (0, 12.1359)
  line L542 (0, 12.1359) -> (3, 13.8679)
  line L543 (3, 13.8679) -> (3, 17.3321)
  line L544 (0, 19.0641) -> (-3, 17.3321)
  line L545 (3, 17.3321) -> (0, 19.0641)
  line L546 (6, 17.3321) -> (6, 13.8679)
  line L547 (6, 13.8679) -> (9, 12.1359)
  line L548 (9, 12.1359) -> (12, 13.8679)
  line L549 (12, 13.8679) -> (12, 17.3321)
  line L550 (9, 19.0641) -> (6, 17.3321)
  line L551 (12, 17.3321) -> (9, 19.0641)
  line L552 (15, 17.3321) -> (15, 13.8679)
  line L553 (15, 13.8679) -> (18, 12.1359)
  line L554 (18, 12.1359) -> (21, 13.8679)
  line L555 (21, 13.8679) -> (21, 17.3321)
  line L556 (18, 19.0641) -> (15, 17.3321)
  line L557 (21, 17.3321) -> (18, 19.0641)
  line L558 (24, 17.3321) -> (24, 13.8679)
  line L559 (24, 13.8679) -> (27, 12.1359)
  line L560 (27, 12.1359) -> (30, 13.8679)
  line L561 (30, 13.8679) -> (30, 17.3321)
  line L562 (27, 19.0641) -> (24, 17.3321)
  line L563 (30, 17.3321) -> (27, 19.0641)
  line L564 (33, 17.3321) -> (33, 13.8679)
  line L565 (33, 13.8679) -> (36, 12.1359)
  line L566 (36, 12.1359) -> (39, 13.8679)
  line L567 (39, 13.8679) -> (39, 17.3321)
  line L568 (36, 19.0641) -> (33, 17.3321)
  line L569 (39, 17.3321) -> (36, 19.0641)
  line L570 (42, 17.3321) -> (42, 13.8679)
  line L571 (42, 13.8679) -> (45, 12.1359)
  line L572 (45, 12.1359) -> (48, 13.8679)
  line L573 (48, 13.8679) -> (48, 17.3321)
  line L574 (45, 19.0641) -> (42, 17.3321)
  line L575 (48, 17.3321) -> (45, 19.0641)
  line L576 (-34.5, 25.1321) -> (-34.5, 21.6679)
  line L577 (-34.5, 21.6679) -> (-31.5, 19.9359)
  line L578 (-31.5, 19.9359) -> (-28.5, 21.6679)
  line L579 (-28.5, 21.6679) -> (-28.5, 25.1321)
  line L580 (-31.5, 26.8641) -> (-34.5, 25.1321)
  line L581 (-28.5, 25.1321) -> (-31.5, 26.8641)
  line L582 (-43.5, 25.1321) -> (-43.5, 21.6679)
  line L583 (-43.5, 21.6679) -> (-40.5, 19.9359)
  line L584 (-40.5, 19.9359) -> (-37.5, 21.6679)
  line L585 (-37.5, 21.6679) -> (-37.5, 25.1321)
  line L586 (-40.5, 26.8641) -> (-43.5, 25.1321)
  line L587 (-37.5, 25.1321) -> (-40.5, 26.8641)
  line L588 (-52.5, 25.1321) -> (-52.5, 21.6679)
  line L589 (-52.5, 21.6679) -> (-49.5, 19.9359)
  line L590 (-49.5, 19.9359) -> (-46.5, 21.6679)
  line L591 (-46.5, 21.6679) -> (-46.5, 25.1321)
  line L592 (-49.5, 26.8641) -> (-52.5, 25.1321)
  line L593 (-46.5, 25.1321) -> (-49.5, 26.8641)
  line L594 (-25.5, 25.1321) -> (-25.5, 21.6679)
  line L595 (-25.5, 21.6679) -> (-22.5, 19.9359)
  line L596 (-22.5, 19.9359) -> (-19.5, 21.6679)
  line L597 (-19.5, 21.6679) -> (-19.5, 25.1321)
  line L598 (-22.5, 26.8641) -> (-25.5, 25.1321)
  line L599 (-19.5, 25.1321) -> (-22.5, 26.8641)
  line L600 (-16.5, 25.1321) -> (-16.5, 21.6679)
  line L601 (-16.5, 21.6679) -> (-13.5, 19.9359)
  line L602 (-13.5, 19.9359) -> (-10.5, 21.6679)
  line L603 (-10.5, 21.6679) -> (-10.5, 25.1321)
  line L604 (-13.5, 26.8641) -> (-16.5, 25.1321)
  line L605 (-10.5, 25.1321) -> (-13.5, 26.8641)
  line L606 (-7.5, 25.1321) -> (-7.5, 21.6679)
  line L607 (-7.5, 21.6679) -> (-4.5, 19.9359)
  line L608 (-4.5, 19.9359) -> (-1.5, 21.6679)
  line L609 (-1.5, 21.6679) -> (-1.5, 25.1321)
  line L610 (-4.5, 26.8641) -> (-7.5, 25.1321)
  line L611 (-1.5, 25.1321) -> (-4.5, 26.8641)
  line L612 (1.5, 25.1321) -> (1.5, 21.6679)
  line L613 (1.5, 21.6679) -> (4.5, 19.9359)
  line L614 (4.5, 19.9359) -> (7.5, 21.6679)
  line L615 (7.5, 21.6679) -> (7.5, 25.1321)
  line L616 (4.5, 26.8641) -> (1.5, 25.1321)
  line L617 (7.5, 25.1321) -> (4.5, 26.8641)
  line L618 (10.5, 25.1321) -> (10.5, 21.6679)
  line L619 (10.5, 21.6679) -> (13.5, 19.9359)
  line L620 (13.5, 19.9359) -> (16.5, 21.6679)
  line L621 (16.5, 21.6679) -> (16.5, 25.1321)
  line L622 (13.5, 26.8641) -> (10.5, 25.1321)
  line L623 (16.5, 25.1321) -> (13.5, 26.8641)
  line L624 (19.5, 25.1321) -> (19.5, 21.6679)
  line L625 (19.5, 21.6679) -> (22.5, 19.9359)
  line L626 (22.5, 19.9359) -> (25.5, 21.6679)
  line L627 (25.5, 21.6679) -> (25.5, 25.1321)
  line L628 (22.5, 26.8641) -> (19.5, 25.1321)
  line L629 (25.5, 25.1321) -> (22.5, 26.8641)
  line L630 (28.5, 25.1321) -> (28.5, 21.6679)
  line L631 (28.5, 21.6679) -> (31.5, 19.9359)
  line L632 (31.5, 19.9359) -> (34.5, 21.6679)
  line L633 (34.5, 21.6679) -> (34.5, 25.1321)
  line L634 (31.5, 26.8641) -> (28.5, 25.1321)
  line L635 (34.5, 25.1321) -> (31.5, 26.8641)
  line L636 (37.5, 25.1321) -> (37.5, 21.6679)
  line L637 (37.5, 21.6679) -> (40.5, 19.9359)
  line L638 (40.5, 19.9359) -> (43.5, 21.6679)
  line L639 (43.5, 21.6679) -> (43.5, 25.1321)
  line L640 (40.5, 26.8641) -> (37.5, 25.1321)
  line L641 (43.5, 25.1321) -> (40.5, 26.8641)
  line L642 (46.5, 25.1321) -> (46.5, 21.6679)
  line L643 (46.5, 21.6679) -> (49.5, 19.9359)
  line L644 (49.5, 19.9359) -> (52.5, 21.6679)
  line L645 (52.5, 21.6679) -> (52.5, 25.1321)
  line L646 (49.5, 26.8641) -> (46.5, 25.1321)
  line L647 (52.5, 25.1321) -> (49.5, 26.8641)
  line L648 (-3, -13.8679) -> (-3, -17.3321)
  line L649 (-3, -17.3321) -> (0, -19.0641)
  line L650 (0, -19.0641) -> (3, -17.3321)
  line L651 (3, -17.3321) -> (3, -13.8679)
  line L652 (0, -12.1359) -> (-3, -13.8679)
  line L653 (3, -13.8679) -> (0, -12.1359)
  line L654 (6, -13.8679) -> (6, -17.3321)
  line L655 (6, -17.3321) -> (9, -19.0641)
  line L656 (9, -19.0641) -> (12, -17.3321)
  line L657 (12, -17.3321) -> (12, -13.8679)
  line L658 (9, -12.1359) -> (6, -13.8679)
  line L659 (12, -13.8679) -> (9, -12.1359)
  line L660 (15, -13.8679) -> (15, -17.3321)
  line L661 (15, -17.3321) -> (18, -19.0641)
  line L662 (18, -19.0641) -> (21, -17.3321)
  line L663 (21, -17.3321) -> (21, -13.8679)
  line L664 (18, -12.1359) -> (15, -13.8679)
  line L665 (21, -13.8679) -> (18, -12.1359)
  line L666 (24, -13.8679) -> (24, -17.3321)
  line L667 (24, -17.3321) -> (27, -19.0641)
  line L668 (27, -19.0641) -> (30, -17.3321)
  line L669 (30, -17.3321) -> (30, -13.8679)
  line L670 (27, -12.1359) -> (24, -13.8679)
  line L671 (30, -13.8679) -> (27, -12.1359)
  line L672 (33, -13.8679) -> (33, -17.3321)
  line L673 (33, -17.3321) -> (36, -19.0641)
  line L674 (36, -19.0641) -> (39, -17.3321)
  line L675 (39, -17.3321) -> (39, -13.8679)
  line L676 (36, -12.1359) -> (33, -13.8679)
  line L677 (39, -13.8679) -> (36, -12.1359)
  line L678 (42, -13.8679) -> (42, -17.3321)
  line L679 (42, -17.3321) -> (45, -19.0641)
  line L680 (45, -19.0641) -> (48, -17.3321)
  line L681 (48, -17.3321) -> (48, -13.8679)
  line L682 (45, -12.1359) -> (42, -13.8679)
  line L683 (48, -13.8679) -> (45, -12.1359)
  line L684 (-7.5, -21.6679) -> (-7.5, -25.1321)
  line L685 (-7.5, -25.1321) -> (-4.5, -26.8641)
  line L686 (-4.5, -26.8641) -> (-1.5, -25.1321)
  line L687 (-1.5, -25.1321) -> (-1.5, -21.6679)
  line L688 (-4.5, -19.9359) -> (-7.5, -21.6679)
  line L689 (-1.5, -21.6679) -> (-4.5, -19.9359)
  line L690 (1.5, -21.6679) -> (1.5, -25.1321)
  line L691 (1.5, -25.1321) -> (4.5, -26.8641)
  line L692 (4.5, -26.8641) -> (7.5, -25.1321)
  line L693 (7.5, -25.1321) -> (7.5, -21.6679)
  line L694 (4.5, -19.9359) -> (1.5, -21.6679)
  line L695 (7.5, -21.6679) -> (4.5, -19.9359)
  line L696 (10.5, -21.6679) -> (10.5, -25.1321)
  line L697 (10.5, -25.1321) -> (13.5, -26.8641)
  line L698 (13.5, -26.8641) -> (16.5, -25.1321)
  line L699 (16.5, -25.1321) -> (16.5, -21.6679)
  line L700 (13.5, -19.9359) -> (10.5, -21.6679)
  line L701 (16.5, -21.6679) -> (13.5, -19.9359)
  line L702 (19.5, -21.6679) -> (19.5, -25.1321)
  line L703 (19.5, -25.1321) -> (22.5, -26.8641)
  line L704 (22.5, -26.8641) -> (25.5, -25.1321)
  line L705 (25.5, -25.1321) -> (25.5, -21.6679)
  line L706 (22.5, -19.9359) -> (19.5, -21.6679)
  line L707 (25.5, -21.6679) -> (22.5, -19.9359)
  line L708 (28.5, -21.6679) -> (28.5, -25.1321)
  line L709 (28.5, -25.1321) -> (31.5, -26.8641)
  line L710 (31.5, -26.8641) -> (34.5, -25.1321)
  line L711 (34.5, -25.1321) -> (34.5, -21.6679)
  line L712 (31.5, -19.9359) -> (28.5, -21.6679)
  line L713 (34.5, -21.6679) -> (31.5, -19.9359)
  line L714 (37.5, -21.6679) -> (37.5, -25.1321)
  line L715 (37.5, -25.1321) -> (40.5, -26.8641)
  line L716 (40.5, -26.8641) -> (43.5, -25.1321)
  line L717 (43.5, -25.1321) -> (43.5, -21.6679)
  line L718 (40.5, -19.9359) -> (37.5, -21.6679)
  line L719 (43.5, -21.6679) -> (40.5, -19.9359)
  line L720 (46.5, -21.6679) -> (46.5, -25.1321)
  line L721 (46.5, -25.1321) -> (49.5, -26.8641)
  line L722 (49.5, -26.8641) -> (52.5, -25.1321)
  line L723 (52.5, -25.1321) -> (52.5, -21.6679)
  line L724 (49.5, -19.9359) -> (46.5, -21.6679)
  line L725 (52.5, -21.6679) -> (49.5, -19.9359)
  dimension "d54" = 9
  dimension "d55" = 0
  dimension "d58" = 9
  dimension "d59" = 0
  dimension "d62" = 9
  dimension "d63" = 0
  dimension "d66" = 9
  dimension "d67" = 0
  dimension "d70" = -9
  dimension "d71" = 0
extrude "Extrude3" cut sketch "Sketch6" against normal blind 4
thread "Thread3" "ISO Metric profile 3.0 M3x0.5 M3x0.5 6H" major diameter 3.086 minor diameter 2.529 pitch 0.5 angle 60 modelled right hand crest width 0.1368 on face at (-57.3128, 25.0313, 1.843) crest through (-55.2355, 26, 2.6395) on face at (-57.3128, -26.9687, 1.843) crest through (-55.2355, -26, 2.6395) on face at (8.1259, 14.7418, 2.6667) crest through (9.2645, 16, 3.875) on face at (47.1872, 16.9687, 2.6667) crest through (49.2645, 16, 3.875) on face at (55.6872, -26.9687, 1.843) crest through (57.7645, -26, 2.6395) on face at (55.6872, 25.0313, 1.843) crest through (57.7645, 26, 2.6395)
